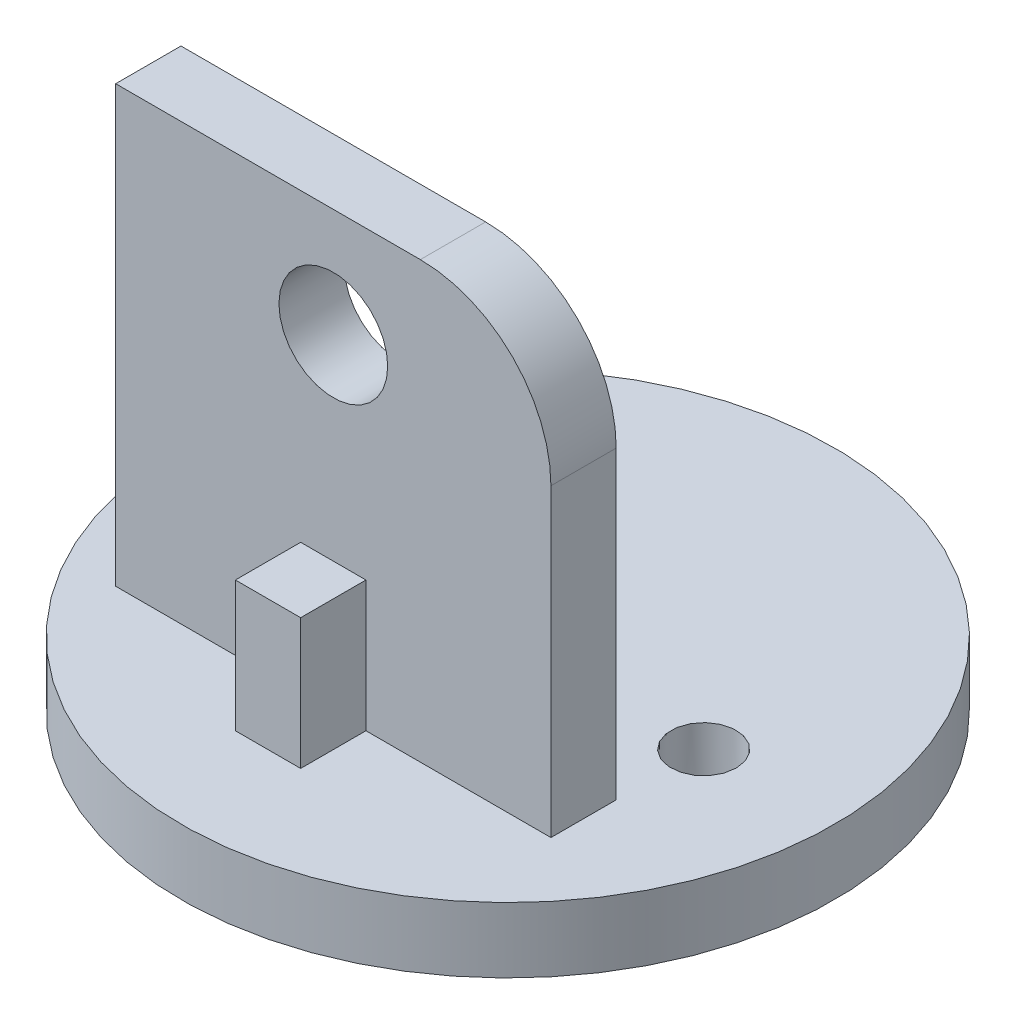
# Autodesk Inventor part: Pad_1
Saved by Autodesk Inventor 2023 (Build 270158000, 158)
## iProperties
Created: 2022-04-08
Part Number: Pad_1
Material: 一般
Document SubType Name: Modeling
Designer: device
Mass: 3.37805 g
Surface Area: 30.7473 cm^2
Volume: 3.37805 cm^3
Density: 1 g/cm^3
Appearance: 預設
Author: device
Autodesk Inventor part; units mm, degrees
ref_plane "YZ Plane" through (0, 0, 0) normal (1, 0, 0) x (0, 1, 0)
ref_plane "XZ Plane" through (0, 0, 0) normal (0, 1, 0) x (-1, 0, 0)
ref_plane "XY Plane" through (0, 0, 0) normal (0, 0, 1) x (1, 0, 0)
sketch "草圖1" plane through (0, 0, 0) normal (0, 1, 0) x (-1, 0, 0)
  circle A0 centre (0, 0) radius 15
  dimension "d0" = 30
  constraints: 1 centre point, 1 coincident
  measures "d0" diameter of A0
extrude "擠出1" add sketch "草圖1" along normal blind 3
sketch "草圖2" plane through (0, 3, 0) normal (0, 1, 0) x (1, 0, 0)
  line L0 (-21, 0) -> (21, 0) construction
  circle A0 centre (-9, 0) radius 1.5
  circle A1 centre (0, 0) radius 1.5
  circle A2 centre (9, 0) radius 1.5
  dimension "d4" = 3
  dimension "d7" = 9
  constraints: 3 centre point, 1 coincident, 1 horizontal, 1 point on line, 4 other
  measures "d4" diameter of A0
  measures "d7" distance of A0.centre A1.centre
extrude "擠出2" cut sketch "草圖2" against normal up to surface (3 mm away)
sketch "草圖3" plane through (0, 3, 0) normal (0, 1, 0) x (1, 0, 0)
  line L0 (-10.9932, -7.0266) -> (9.0068, -7.0266)
  line L1 (9.0068, -7.0266) -> (9.0068, -4.0266)
  line L2 (9.0068, -4.0266) -> (-10.9932, -4.0266)
  line L3 (-10.9932, -4.0266) -> (-10.9932, -7.0266)
  point P0 (0, 0)
  dimension "d14" = 20
  dimension "d15" = 3
  constraints: 8 end point, 2 parallel, 1 horizontal, 1 perpendicular
  measures "d14" distance of L2.end L1.end
  measures "d15" distance of L1.end L0.end
extrude "擠出3" add sketch "草圖3" along normal blind 20 separate body
sketch "草圖4" plane through (-10.9932, 3, 7.0266) normal (0, 0, 1) x (1, 0, 0)
  line L0 (20, 0) -> (0, 0) construction
  line L1 (20, 0) -> (20, 20) construction
  line L2 (0, 20) -> (20, 20) construction
  line L3 (0, 0) -> (0, 20) construction
  line L4 (0, 20) -> (10, 20) construction
  line L5 (10, 20) -> (10, 15) construction
  line L6 (10, 15) -> (0, 15) construction
  line L7 (0, 15) -> (0, 20) construction
  circle A0 centre (10, 15) radius 2.5
  point P0 (10.9932, -3)
  dimension "d18" = 15
  dimension "d19" = 5
  constraints: 8 end point, 2 parallel, 1 centre point, 1 coincident, 1 horizontal, 1 midpoint, 1 perpendicular
  measures "d18" distance between parallel lines of L0 L6
  measures "d19" diameter of A0
extrude "擠出4" cut sketch "草圖4" against normal up to surface (3 mm away) bodies 2
sketch "草圖5" plane through (0, 0, 0) normal (0, -1, 0) x (1, 0, 0)
  line L0 (0.5068, 10.0266) -> (-2.4932, 10.0266)
  line L1 (-2.4932, 10.0266) -> (-2.4932, 4.0266)
  line L2 (-2.4932, 4.0266) -> (0.5068, 4.0266)
  line L3 (0.5068, 4.0266) -> (0.5068, 10.0266)
  line L4 (9.0068, 7.0266) -> (9.0068, 4.0266) projected
  line L5 (9.0068, 4.0266) -> (-10.9932, 4.0266) projected
  line L6 (-10.9932, 4.0266) -> (-10.9932, 7.0266) projected
  line L7 (-10.9932, 7.0266) -> (9.0068, 7.0266) projected
  point P0 (0, 0)
  point P1 (-0.9932, 4.0266)
  dimension "d22" = 6
  constraints: 8 end point, 2 midpoint, 2 parallel, 2 perpendicular, 1 horizontal
  measures "d22" distance of L0.end L1.end
extrude "擠出5" cut sketch "草圖5" against normal blind 9 contours L3 L7 L1 L0 | L3 L2 L1 L7 bodies 1
extrude "擠出6" add sketch "草圖5" against normal blind 9 separate body contours L3 L7 L1 L0 | L3 L2 L1 L7
fillet "圓角1" radius 6 1 edges at (9.0068, 23, 5.5266)
equation "\"d16\" = d14"
